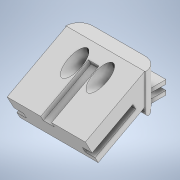
# Autodesk Inventor part: bottomclip
Saved by Autodesk Inventor 2020 (Build 240168000, 168)
## iProperties
Created: 2020-12-04
Part Number: bottomclip
Material: Generic
Document SubType Name: Modeling
Designer: Curtis
Density: 1 g/cm^3
Appearance: Default
Author: Curtis
Autodesk Inventor part; units mm, degrees
ref_plane "YZ Plane" through (0, 0, 0) normal (1, 0, 0) x (0, 1, 0)
ref_plane "XZ Plane" through (0, 0, 0) normal (0, 1, 0) x (-1, 0, 0)
sketch "Sketch1" plane through (0, 0, 0) normal (0, 1, 0) x (-1, 0, 0)
  line L0 (0, 0) -> (15, 0)
  line L1 (15, 0) -> (15, -29.5)
  line L2 (15, -29.5) -> (0, -29.5)
  line L3 (0, -29.5) -> (0, 0)
  dimension "d0" = 15
  dimension "d1" = 29.5
  constraints: 8 end point, 2 parallel, 1 horizontal, 1 perpendicular
  measures "d0" distance of L1.end L2.end
  measures "d1" distance of L0.end L1.end
extrude "Extrusion1" add sketch "Sketch1" along normal blind 5
fillet "Fillet1" radius 5 2 edges at (-7.5, 5, 0) (-7.5, 5, -29.5)
sketch "Sketch2" plane through (0, 0, 0) normal (0, -1, 0) x (1, 0, 0)
  circle A0 centre (-3.581, -10) radius 1.5
  line L0 (-15, -29.5) -> (-15, 0) projected
  line L1 (-15, -14.75) -> (-4.074, -14.75)
  line L2 (-4.074, 0) -> (-4.074, -29.5) projected
  circle A1 centre (-3.581, -19.5) radius 1.5
  line L3 (0, -27.3987) -> (0, -2.1013) projected
  point P0 (0, 0)
  dimension "d6" = 3
  dimension "d7" = 4.75
  dimension "d8" = 10.926
  dimension "d10" = 3
  dimension "d11" = 4.75
  dimension "d15" = 3.581
  dimension "d16" = 3.581
  constraints: 2 centre point, 2 end point, 2 midpoint
  measures "d6" diameter of A0
  measures "d7" distance from line of L1 A0.centre
  measures "d8" distance between parallel lines of L0 L2
  measures "d10" diameter of A1
  measures "d11" distance from line of L1 A1.centre
  measures "d15" distance from line of L3 A0.centre
  measures "d16" distance from line of L3 A1.centre
extrude "Extrusion2" cut sketch "Sketch2" against normal up to surface (5 mm away)
fillet "Fillet3" radius 1.993 1 edges at (-15, 0, -14.75)
sketch "Sketch3" plane through (0, 0, 0) normal (0, -1, 0) x (1, 0, 0)
  circle A0 centre (-3.581, -10) radius 2.5
  circle A1 centre (-3.581, -19.5) radius 2.5
  circle A2 centre (-3.581, -10) radius 1.5 projected
  circle A3 centre (-3.581, -19.5) radius 1.5 projected
  point P0 (0, 0)
  dimension "d18" = 5
  dimension "d19" = 5
  dimension "d20" = 0
  dimension "d21" = 0
  dimension "d22" = 0
  dimension "d23" = 0
  constraints: 2 centre point
  measures "d18" diameter of A0
  measures "d19" diameter of A1
  measures "d20" distance of A2.centre A0.centre
  measures "d21" distance of A2.centre A0.centre
  measures "d22" distance of A3.centre A1.centre
  measures "d23" distance of A3.centre A1.centre
extrude "Extrusion3" cut sketch "Sketch3" along normal blind 32.5 and the other way blind 0.375
sketch "Sketch4" plane through (-15, 5, -24.5) normal (-1, 0, 0) x (0, 0, 1)
  line L0 (24.5, -3.007) -> (-5, -3.007)
  line L1 (-5, -3.007) -> (-5, 0)
  line L2 (-5, 0) -> (24.5, 0)
  line L3 (24.5, 0) -> (24.5, -3.007)
  line L4 (-5, -5) -> (24.5, -5) projected
  line L5 (0, 0) -> (19.5, 0) projected
  dimension "d26" = 1.993
  dimension "d27" = 0
  dimension "d28" = 0
  dimension "d29" = 0
  constraints: 8 end point, 2 parallel, 1 horizontal, 1 perpendicular
  measures "d26" distance between parallel lines of L4 L0
  measures "d27" distance from line of L4.end L3
  measures "d28" distance from line of L4.start L1
  measures "d29" distance between parallel lines of L5 L2
extrude "Extrusion4" add sketch "Sketch4" against normal blind 4.356
sketch "Sketch6" plane through (-15, 1.993, -29.5) normal (0, 0, -1) x (-1, 0, 0)
  line L0 (-3.661, 2.484) -> (-3.051, 2.484)
  line L1 (-0.856, 2.484) -> (-0.856, 8.484)
  line L2 (-0.856, 8.484) -> (-5.856, 8.484)
  line L3 (-5.856, 8.484) -> (-5.856, 2.484)
  line L4 (-15, -1.993) -> (-1.993, -1.993) projected
  line L5 (0, 3.007) -> (0, 0) projected
  line L6 (-15, -1.993) -> (-15, 3.007) projected
  line L7 (-4.356, 8.484) -> (-4.356, 3.179)
  line L8 (-2.356, 8.484) -> (-2.356, 3.179)
  arc A0 (-4.356, 3.179) -> (-3.661, 2.484) centre (-3.661, 3.179) ccw
  arc A1 (-3.051, 2.484) -> (-2.356, 3.179) centre (-3.051, 3.179) ccw
  line L9 (-0.856, 2.484) -> (-3.051, 2.484)
  line L10 (-5.856, 2.484) -> (-3.661, 2.484)
  line L11 (-5.856, 2.484) -> (-7.856, 2.484)
  line L12 (-15, 3.007) -> (-4.356, 3.007) projected
  line L13 (-5.856, 2.484) -> (-3.856, 2.484) construction
  line L14 (-7.856, 2.484) -> (-7.856, 8.484)
  line L15 (-7.856, 3.3104) -> (-5.856, 3.3104)
  point P0 (-10.926, -1.993)
  point P1 (-4.356, -1.993)
  dimension "d37" = 4.477
  dimension "d38" = 0.856
  dimension "d39" = 10.477
  dimension "d40" = 9.144
  dimension "d41" = 1.5
  dimension "d42" = 1.5
  dimension "d43" = 2
  dimension "d44" = 0.695
  dimension "d45" = 2
  dimension "d46" = 180
  constraints: 24 end point, 6 point on line, 6 tangent, 5 perpendicular, 4 point on circle, 3 horizontal, 3 parallel, 2 centre point, 2 collinear, 1 equal radius
  measures "d37" distance between parallel lines of L4 L0
  measures "d38" distance between parallel lines of L5 L1
  measures "d39" distance between parallel lines of L4 L2
  measures "d40" distance between parallel lines of L6 L3
  measures "d41" distance between parallel lines of L7 L3
  measures "d42" distance between parallel lines of L1 L8
  measures "d43" distance between parallel lines of L8 L7
  measures "d44" radius of A0
  measures "d45" distance of L3.end L11.end
  measures "d46" angle of L13 L11
extrude "Extrusion6" cut sketch "Sketch6" against normal up to surface (29.5 mm away)
extrude "Extrusion7" add sketch "Sketch6" against normal up to surface (29.5 mm away) contours L10 L3 L2 L7 A0 | A1 L8 L2 L1 L9
extrude "Extrusion8" cut sketch "Sketch6" against normal blind 2.774 contours L10 L3 L2 L7 A0 | A1 L8 L2 L1 L9
sketch "Sketch7" plane through (-15, 1.993, 0) normal (0, 0, 1) x (1, 0, 0)
  line L0 (5.856, 8.484) -> (5.856, 2.484) projected
  line L1 (5.856, 2.484) -> (0.856, 2.484)
  line L2 (0.856, 2.484) -> (0.856, 11.6469)
  line L3 (0.856, 11.6469) -> (5.856, 11.6469)
  line L4 (5.856, 11.6469) -> (5.856, 2.484)
  line L5 (0.856, 3.007) -> (0.856, 8.484) projected
  point P0 (15, -1.993)
  dimension "d53" = 0
  constraints: 8 end point, 2 parallel, 1 horizontal, 1 perpendicular
  measures "d53" distance between parallel lines of L5 L2
extrude "Extrusion9" cut sketch "Sketch7" against normal blind 2.774
sketch "Sketch8" plane through (-10.644, 5, -24.5) normal (1, 0, 0) x (0, 0, -1)
  arc A0 (4.5856, -3.007) -> (2.2263, -0.523) centre (0, -5) ccw projected
  arc A1 (4.5856, -3.007) -> (2.2263, -0.523) centre (0, -5) ccw
  line L0 (4.5856, -3.007) -> (5, -3.007) projected
  line L1 (4.5856, -3.007) -> (5, -3.007)
  line L2 (5, -3.007) -> (5, -0.523) projected
  line L3 (5, -3.007) -> (5, -0.523)
  line L4 (-24.5, 0) -> (5, 0) projected
  line L5 (5, -0.523) -> (5, 0)
  line L6 (5, 0) -> (2.226, 0)
  line L7 (2.226, -0.523) -> (2.226, 5.477) projected
  line L8 (2.226, -0.523) -> (2.226, 0)
  arc A2 (-19.5, 0) -> (-24.5, -5) centre (-19.5, -5) ccw projected
  line L9 (-24.0856, -3.007) -> (4.5856, -3.007) projected
  arc A3 (-21.7263, -0.523) -> (-24.0856, -3.007) centre (-19.5, -5) ccw
  line L10 (-24.5, -3.007) -> (-24.0856, -3.007) projected
  line L11 (-24.0856, -3.007) -> (-24.5, -3.007)
  line L12 (-24.5, -3.007) -> (-24.5, 0)
  line L13 (-24.5, 0) -> (-21.7263, 0)
  line L14 (2.2263, -0.523) -> (-21.7263, -0.523) projected
  line L15 (-21.7263, -0.523) -> (-21.7263, 0)
  line L16 (-21.726, 5.477) -> (-21.726, -0.523) projected
  point P0 (-22.3987, -0.926)
  point P1 (-24.0856, -3.007)
  point P2 (2.226, 0)
  constraints: 18 end point, 5 point on circle, 3 collinear, 2 centre point, 2 perpendicular, 2 point on line, 1 horizontal, 1 parallel
extrude "Extrusion10" cut sketch "Sketch8" against normal blind 9.726 contours A0 L7 L4 L5 L2 L0 | L10 L12 L4 L15 A2
ref_plane "Work Plane1" through (-11.25, 0, 0) normal (0, 0, 1) x (1, 0, 0)
sketch "Sketch9" plane through (-11.25, 0, 0) normal (0, 0, 1) x (1, 0, 0)
  line L0 (11.25, 0) -> (-1.757, 0) projected
  line L1 (11.25, 0) -> (17.6322, 0) construction
  line L2 (11.25, 0) -> (6.4097, 2.5736)
  line L3 (6.4097, 2.5736) -> (-5.3271, -19.5)
  line L4 (-5.3271, -19.5) -> (-0.4868, -22.0737)
  line L5 (-0.4868, -22.0737) -> (11.25, 0)
  line L6 (11.25, 0) -> (15.8244, 0)
  point P0 (5.0413, 0)
  dimension "d59" = 5.482
  dimension "d60" = 25
  dimension "d61" = 118
  dimension "d62" = 0
  dimension "d63" = 0
  constraints: 12 end point, 2 parallel, 1 horizontal, 1 perpendicular, 1 point on line
  measures "d59" distance of L4.end L3.end
  measures "d60" distance of L3.end L2.end
  measures "d61" angle of L1 L5
  measures "d62" distance from line of L0 L2.start
  measures "d63" distance of L0.start L2.start
extrude "Extrusion11" add sketch "Sketch9" against normal blind 29.5 contours L5 L4 L3 L0
sketch "Sketch10" plane through (-16.5771, -19.5, -29.5) normal (-0.4694716, -0.8829476, 0) x (0.8829476, -0.4694716, 0)
  line L0 (5.482, 29.2875) -> (0, 29.2875)
  line L1 (0, 29.2875) -> (0, 0.2125)
  line L2 (0, 0.2125) -> (5.482, 0.2125)
  line L3 (5.482, 0.2125) -> (5.482, 29.2875)
  line L4 (5.482, 29.5) -> (5.482, 0) projected
  line L5 (0, 29.5) -> (0, 0) projected
  line L6 (5.482, 0) -> (0, 0) projected
  line L7 (0, 29.5) -> (5.482, 29.5) projected
  point P0 (5.482, 0.2125)
  point P1 (0, 0.2125)
  point P2 (0, 29.2875)
  point P3 (5.482, 29.2875)
  dimension "d66" = 0
  dimension "d67" = 0
  dimension "d68" = 0.2125
  dimension "d69" = 0.2125
  dimension "d70" = 29.075
  constraints: 8 end point, 2 parallel, 1 horizontal, 1 perpendicular
  measures "d66" distance between parallel lines of L4 L3
  measures "d67" distance between parallel lines of L5 L1
  measures "d68" distance between parallel lines of L6 L2
  measures "d69" distance between parallel lines of L7 L0
  measures "d70" distance of L2.end L0.start
extrude "Extrusion12" cut sketch "Sketch10" against normal up to surface contours L0 L5 L7 L4 | L4 L6 L5 L2 surface through (-7.5, 0, -14.75) normal (0, 1, 0)
sketch "Sketch11" plane through (-11.7368, -22.0737, -29.2875) normal (-0.4694716, -0.8829476, 0) x (0.8829476, -0.4694716, 0)
  line L0 (-5.482, 0) -> (-5.482, 29.075) projected
  line L1 (0, 0) -> (-5.482, 0) projected
  line L2 (-5.482, 29.075) -> (-5.382, 29.075)
  line L3 (-5.382, 29.075) -> (-5.382, 0)
  line L4 (-5.382, 0) -> (-5.482, 0)
  line L5 (-5.482, 0) -> (-5.482, 29.075)
  point P0 (0, 29.2875)
  dimension "d73" = 0.1
  constraints: 8 end point, 2 parallel, 1 horizontal, 1 perpendicular, 1 point on line
  measures "d73" distance of L3.end L4.end
extrude "Extrusion13" cut sketch "Sketch11" against normal up to surface surface through (-7.5, 0, -14.75) normal (0, 1, 0)
sketch "Sketch12" plane through (-16.4888, -19.547, -29.2875) normal (-0.8829476, 0.4694716, 0) x (0, 0, 1)
  line L0 (25.519, 0) -> (3.556, 0)
  line L1 (3.556, 0) -> (3.556, 17.1383)
  line L2 (3.556, 17.1383) -> (25.519, 17.1383)
  line L3 (25.519, 17.1383) -> (25.519, 0)
  line L4 (29.075, 0) -> (0, 0) projected
  line L5 (0, 0) -> (0, 22.1383) projected
  line L6 (0, 22.1383) -> (29.075, 22.1383) projected
  line L7 (29.075, 22.1383) -> (29.075, 0) projected
  line L8 (29.075, 17.1383) -> (0, 17.1383)
  line L9 (0, 17.1383) -> (0, 22.1383)
  line L10 (0, 22.1383) -> (29.075, 22.1383)
  line L11 (29.075, 22.1383) -> (29.075, 17.1383)
  point P0 (29.2875, 25)
  point P1 (3.556, 17.1383)
  point P2 (25.519, 17.1383)
  dimension "d76" = 0
  dimension "d77" = 21.963
  dimension "d78" = 29.075
  dimension "d79" = 3.556
  dimension "d80" = 5
  constraints: 16 end point, 4 parallel, 2 horizontal, 2 perpendicular, 2 point on line
  measures "d76" distance between parallel lines of L4 L0
  measures "d77" distance of L1.end L2.end
  measures "d78" distance of L4.start L4.end
  measures "d79" distance between parallel lines of L5 L1
  measures "d80" distance between parallel lines of L6 L2
extrude "Extrusion14" add sketch "Sketch12" along normal blind 2.342 contours L0 L1 L2 L3 | L2 L8 L5 L6 L7
sketch "Sketch13" plane through (-18.5567, -18.4475, -29.2875) normal (-0.8829476, 0.4694716, 0) x (0, 0, 1)
  line L0 (0, 20.8931) -> (29.075, 20.8931) projected
  line L1 (29.075, 0) -> (0, 0)
  line L2 (0, 0) -> (0, 20.8931)
  line L3 (0, 20.8931) -> (29.075, 20.8931)
  line L4 (29.075, 20.8931) -> (29.075, 0)
  point P0 (29.2875, 25)
  point P1 (29.075, 20.8931)
  constraints: 8 end point, 2 parallel, 1 horizontal, 1 perpendicular
extrude "Extrusion15" add sketch "Sketch13" along normal blind 2.5
sketch "Sketch14" plane through (-11.7368, -22.0737, -29.2875) normal (-0.4694716, -0.8829476, 0) x (0.8829476, -0.4694716, 0)
  line L0 (0, 16.5425) -> (-2.05, 16.5425)
  line L1 (-2.05, 16.5425) -> (-2.05, 12.5325)
  line L2 (-2.05, 12.5325) -> (0, 12.5325)
  line L3 (0, 12.5325) -> (0, 16.5425)
  line L4 (0, 29.075) -> (0, 0) projected
  line L5 (-5.382, 0) -> (0, 0) projected
  point P0 (0, 29.2875)
  dimension "d85" = 0
  dimension "d86" = 4.01
  dimension "d87" = 29.075
  dimension "d88" = 12.5325
  dimension "d89" = 2.05
  constraints: 8 end point, 2 parallel, 1 horizontal, 1 perpendicular
  measures "d85" distance between parallel lines of L4 L3
  measures "d86" distance between parallel lines of L0 L2
  measures "d87" distance of L4.start L4.end
  measures "d88" distance between parallel lines of L5 L2
  measures "d89" distance of L1.end L2.end
extrude "Extrusion16" cut sketch "Sketch14" against normal blind 20
extrude "Extrusion17" cut sketch "Sketch3" along normal blind 32.5 contours A0 | A1 | A2 | A3
body "Solid1"
